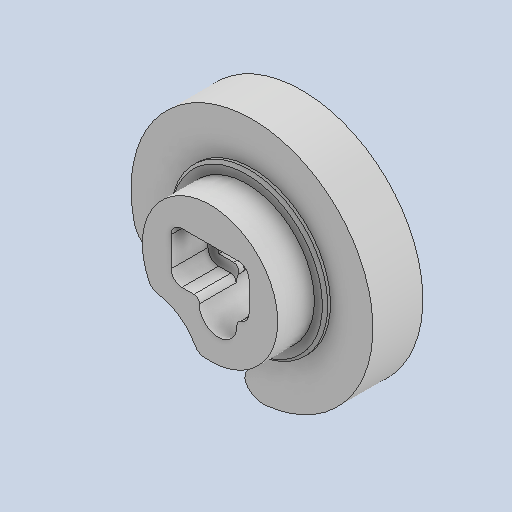
# Autodesk Inventor part: main_wheel_fixator
Saved by Autodesk Inventor 2022 (Build 260153000, 153)
## iProperties
Created: 2024-09-10
Part Number: main_wheel_fixator
Material: Типовые
Document SubType Name: Modeling
Designer: Andrey
Density: 1 g/cm^3
Appearance: По умолчанию
Author: Andrey
Autodesk Inventor part; units mm, degrees
ref_plane "YZ Plane" through (0, 0, 0) normal (1, 0, 0) x (0, 1, 0)
ref_plane "XZ Plane" through (0, 0, 0) normal (0, 1, 0) x (-1, 0, 0)
ref_plane "XY Plane" through (0, 0, 0) normal (0, 0, 1) x (1, 0, 0)
ref_plane "РабПлоскость1" through (-130.0323, -33.3842, -9.2947) normal (0, 0, 1) x (1, 0, 0)
sketch "Эскиз1" plane through (0, 0, 0) normal (0, 0, 1) x (1, 0, 0)
  circle A0 centre (0, 0) radius 22.5
  dimension "d0" = 45
  constraints: 1 centre point, 1 coincident
  measures "d0" diameter of A0
extrude "Выдавливание1" add sketch "Эскиз1" against normal up to surface (9.2947 mm away)
sketch "Эскиз2" plane through (0, 0, 0) normal (0, 0, 1) x (1, 0, 0)
  arc A0 (-12.5314, -17.4431) -> (-12.5619, -14.5867) centre (-11.1467, -16) ccw projected
  circle A1 centre (-11.1467, -16) radius 6.5
  circle A2 centre (-11.1467, -16) radius 9.5
  point P0 (0, 0)
  dimension "d3" = 13
  dimension "d4" = 3
  constraints: 2 centre point, 1 coincident
  measures "d3" diameter of A1
  measures "d4" radial gap between concentric circles of A1 A2
extrude "Выдавливание2" cut sketch "Эскиз2" against normal blind 10 contours A1 | A2
fillet "Сопряжение1" radius 4 2 edges at (-3.9122, -22.1573, -4.6474) (-19.4292, -11.347, -4.6474)
sketch "Эскиз3" plane through (0, 0, 0) normal (0, 0, 1) x (1, 0, 0)
  circle A0 centre (0, 0) radius 12.6
  arc A1 (-21.8671, -5.2989) -> (-15.9551, -7.8067) centre (-17.9796, -4.3569) ccw projected
  arc A2 (-1.795, -17.6717) -> (-15.9551, -7.8067) centre (-11.1467, -16) ccw projected
  arc A3 (-1.795, -17.6717) -> (2.6059, -22.3486) centre (2.1426, -18.3755) ccw projected
  arc A4 (2.6059, -22.3486) -> (-21.8671, -5.2989) centre (0, 0) ccw projected
  line L0 (0, 0) -> (0, -1.1)
  line L1 (5, 3.9) -> (-5, 3.9)
  line L2 (-5, 3.9) -> (-5, -1.1)
  line L3 (-5, -1.1) -> (5, -1.1)
  line L4 (5, -1.1) -> (5, 3.9)
  line L5 (5.25, -1.35) -> (-5.25, -1.35)
  line L6 (-5.25, -1.35) -> (-5.25, 4.15)
  line L7 (-5.25, 4.15) -> (5.25, 4.15)
  line L8 (5.25, 4.15) -> (5.25, -1.35)
  point P0 (-10.7899, -6.5067)
  point P1 (-2.3651, -12.376)
  dimension "d8" = 25.2
  dimension "d35" = 1.1
  dimension "d36" = 10
  dimension "d37" = 5
  dimension "d38" = 0.25
  constraints: 18 end point, 4 parallel, 2 coincident, 2 perpendicular, 1 centre point, 1 horizontal, 1 midpoint, 1 vertical, 3 other
  measures "d8" diameter of A0
  measures "d35" distance of L0.end L0.start
  measures "d36" distance of L3.end L2.end
  measures "d37" distance of L2.end L1.end
  measures "d38" distance between parallel lines of L3 L5
extrude "Выдавливание3" add sketch "Эскиз3" along normal blind 7.8 contours A0 A2 picked at (0.4072, 6.9469)
sketch "Эскиз4" plane through (0, 0, 0) normal (0, 0, 1) x (1, 0, 0)
  arc A0 (-2.3651, -12.376) -> (-10.7899, -6.5067) centre (0, 0) ccw projected
  arc A1 (-1.795, -17.6717) -> (-2.3651, -12.376) centre (-11.1467, -16) ccw projected
  arc A2 (-1.795, -17.6717) -> (2.6059, -22.3486) centre (2.1426, -18.3755) ccw projected
  arc A3 (2.6059, -22.3486) -> (-21.8671, -5.2989) centre (0, 0) ccw projected
  arc A4 (-21.8671, -5.2989) -> (-15.9551, -7.8067) centre (-17.9796, -4.3569) ccw projected
  arc A5 (-10.7899, -6.5067) -> (-15.9551, -7.8067) centre (-11.1467, -16) ccw projected
  circle A6 centre (0, 0) radius 12.6
  circle A7 centre (0, 0) radius 14.6
  point P0 (-1.7671, -14.4927)
  point P1 (-12.9827, -6.6791)
  dimension "d13" = 2
  constraints: 2 centre point, 1 coincident, 1 concentric
  measures "d13" radial gap between concentric circles of A6 A7
extrude "Выдавливание4" add sketch "Эскиз4" along normal blind 1 contours A0 A5 A7 A1
fillet "Сопряжение2" radius 2 4 edges at (-2.3651, -12.376, 4.4) (-1.7671, -14.4927, 0.5) (-10.7899, -6.5067, 4.4) (-12.9827, -6.6791, 0.5)
chamfer "Фаска1" distance 0.5 angle 45 7 edges at (8.3458, 11.9795, 1) (-12.8509, -6.1946, 1) (-11.2228, -6.5003, 1) (-10.3052, -6.5373, 1) (-1.3582, -14.2012, 1) (-2.2091, -12.7799, 1) (-2.5618, -11.932, 1)
sketch "Эскиз5" plane through (0, 0, -9.2947) normal (0, 0, -1) x (-0.8205128, 0.5716281, 0)
  circle A0 centre (-6.9744, -14.6412) radius 1.5
  arc A1 (5.5942, -23.7713) -> (7.8344, -23.1299) centre (6.9744, -24.3588) ccw
  arc A2 (5.5942, -23.7713) -> (5.8702, -23.7046) centre (0, 0) ccw
  spline S0 degree 3 poles (7.0407, -25.2882) (6.986, -25.2268) (6.8766, -25.1041) (6.7176, -24.9155) (6.5628, -24.7236) (6.4128, -24.5278) (6.2678, -24.3283) (6.1284, -24.1248) (6.0175, -23.9518) (5.9319, -23.8114) (5.8908, -23.7402) (5.8702, -23.7046) knots 0 0 0 0 0.125 0.250001 0.375002 0.500002 0.625001 0.75 0.874998 0.937499 1 1 1 1
  arc A3 (7.0407, -25.2882) -> (7.5579, -25.1384) centre (0, 0) ccw
  spline S1 degree 3 poles (7.7014, -23.1745) (7.703, -23.2156) (7.7063, -23.2977) (7.709, -23.4621) (7.7076, -23.6676) (7.6985, -23.9141) (7.6826, -24.1602) (7.6603, -24.4058) (7.632, -24.6508) (7.5984, -24.8952) (7.5714, -25.0573) (7.5579, -25.1384) knots 0 0 0 0 0.062501 0.125002 0.25 0.374999 0.499998 0.624998 0.749999 0.875 1 1 1 1
  arc A4 (7.7014, -23.1745) -> (7.8344, -23.1299) centre (0, 0) ccw
  circle A5 centre (0, -19.5) radius 4.5
  line L0 (-92.3726, 48.2814) -> (-109.8668, 39.9786)
  line L1 (13.2101, -45.7656) -> (-109.8668, 39.9786)
  line L2 (13.2101, -45.7656) -> (14.9372, -26.4783)
  arc A6 (18.1683, -19.9728) -> (14.9372, -26.4783) centre (24.8973, -27.3701) ccw
  arc A7 (18.1683, -19.9728) -> (-19.7633, 18.396) centre (0, 0) ccw
  arc A8 (-26.2813, 17.7001) -> (-19.7633, 18.396) centre (-23.4232, 21.8026) ccw
  line L3 (-26.2813, 17.7001) -> (-36.6493, 24.9232)
  arc A9 (-38.2549, 31.2785) -> (-36.6493, 24.9232) centre (-33.7911, 29.0257) ccw
  arc A10 (-38.2549, 31.2785) -> (-87.3896, 53.5664) centre (-62.359, 43.4437) ccw
  arc A11 (-92.3726, 48.2814) -> (-87.3896, 53.5664) centre (-96.6602, 57.3156) ccw
  circle A12 centre (-4.5825, 16.9412) radius 2.1
  circle A13 centre (10.0321, 14.4) radius 2.1
  circle A14 centre (17.4795, 1.5711) radius 2.1
  circle A15 centre (10.0321, 14.4) radius 3.5
  circle A16 centre (-4.5825, 16.9412) radius 3.5
  circle A17 centre (17.4795, 1.5711) radius 3.5
  circle A18 centre (-52.3269, 57.8437) radius 3.5
  circle A19 centre (-44.8794, 45.0149) radius 3.5
  circle A20 centre (-66.9415, 60.3849) radius 3.5
  circle A21 centre (-63.7005, 38.894) radius 1.5
  circle A22 centre (-3.8031, -2.8349) radius 1.5
  circle A23 centre (-39.8968, 9.209) radius 1.5
  point P0 (0, 0)
  dimension "d20" = 4.2
  dimension "d21" = 4.2
  dimension "d22" = 4.2
  constraints: 3 centre point
  measures "d20" diameter of A12
  measures "d21" diameter of A13
  measures "d22" diameter of A14
extrude "Выдавливание5" cut sketch "Эскиз5" against normal blind 7.5 contours A12 | A13 | A14
sketch "Эскиз6" plane through (0, 0, 7.8) normal (0, 0, 1) x (1, 0, 0)
  circle A0 centre (1.5, -4.5) radius 1.5 projected
  circle A1 centre (1.5, -4.5) radius 1.6
  point P0 (0, 0)
  dimension "d25" = 3.2
  constraints: 1 centre point, 1 coincident
  measures "d25" diameter of A1
extrude "Выдавливание6" cut sketch "Эскиз6" against normal blind 20 contours A0 | A1
sketch "Эскиз7" plane through (0, 0, 7.8) normal (0, 0, 1) x (1, 0, 0)
  circle A0 centre (1.5, -4.5) radius 1.5 projected
  circle A1 centre (1.5, -4.5) radius 3.5
  point P0 (0, 0)
  dimension "d28" = 7
  constraints: 1 centre point, 1 coincident
  measures "d28" diameter of A1
extrude "Выдавливание7" cut sketch "Эскиз7" against normal blind 13 contours A0 | A1
sketch "Эскиз9" plane through (0, 0, 7.8) normal (0, 0, 1) x (1, 0, 0)
  arc A0 (-0.0256, -1.35) -> (3.0256, -1.35) centre (1.5, -4.5) ccw projected
  line L0 (-0.0256, -1.35) -> (-5.25, -1.35) projected
  line L1 (-5.25, -1.35) -> (-5.25, 4.15) projected
  line L2 (-5.25, 4.15) -> (5.25, 4.15) projected
  line L3 (5.25, 4.15) -> (5.25, -1.35) projected
  line L4 (5.25, -1.35) -> (3.0256, -1.35) projected
  arc A1 (-11.3447, -5.4825) -> (-9.8227, -6.5927) centre (-9.544, -4.6122) ccw projected
  arc A2 (-2.7809, -11.4985) -> (-9.8227, -6.5927) centre (-11.1467, -16) ccw projected
  arc A3 (-2.7809, -11.4985) -> (-1.2121, -12.5416) centre (-1.0197, -10.5508) ccw projected
  arc A4 (-1.2121, -12.5416) -> (-11.3447, -5.4825) centre (0, 0) ccw projected
  arc A5 (-3.8784, -3.35) -> (6.8784, -3.35) centre (1.5, -4.5) ccw
  line L5 (-3.8784, -3.35) -> (-7.25, -3.35)
  line L6 (-7.25, -3.35) -> (-7.25, 6.15)
  line L7 (-7.25, 6.15) -> (7.25, 6.15)
  line L8 (7.25, 6.15) -> (7.25, -3.35)
  line L9 (7.25, -3.35) -> (6.8784, -3.35)
  line L10 (7.25, -3.35) -> (-7.25, -3.35)
  point P0 (4.8057, -3.35)
  point P1 (6.8784, -3.35)
  point P2 (-1.8057, -3.35)
  dimension "d39" = 2
  constraints: 12 end point, 2 point on circle, 1 centre point, 1 collinear, 5 other
  measures "d39" distance between parallel lines of L4 L9
extrude "Выдавливание9" cut sketch "Эскиз9" against normal blind 6.85 contours A0 L10 L5 L6 L7 L8 L9 L4 L3 L2 L1 L0
fillet "Сопряжение3" radius 2 4 edges at (7.25, -3.35, 4.375) (-7.25, -3.35, 4.375) (-7.25, 6.15, 4.375) (7.25, 6.15, 4.375)
fillet "Сопряжение4" radius 1 4 edges at (-1.8057, -3.35, 4.375) (4.8057, -3.35, 4.375) (3.0256, -1.35, 0.475) (-0.0256, -1.35, 0.475)
sketch "Эскиз10" plane through (0, 0, 0) normal (0, 0, 1) x (1, 0, 0)
  circle A0 centre (-2.6467, -16) radius 1.5 projected
  circle A1 centre (-19.6467, -16) radius 1.5 projected
  line L0 (55, -39.3) -> (55, -42.3) projected
  line L1 (55, -42.3) -> (47, -42.3) projected
  line L2 (47, -42.3) -> (47, -39.3) projected
  line L3 (47, -39.3) -> (55, -39.3) projected
  line L4 (29, -39.3) -> (29, -42.3) projected
  line L5 (29, -42.3) -> (21, -42.3) projected
  line L6 (21, -42.3) -> (21, -39.3) projected
  line L7 (21, -39.3) -> (29, -39.3) projected
  arc A2 (56, -45.3) -> (59, -42.3) centre (56, -42.3) ccw projected
  line L8 (59, -42.3) -> (59, -31) projected
  arc A3 (60, -30) -> (59, -31) centre (60, -31) ccw projected
  line L9 (117, -30) -> (60, -30) projected
  line L10 (106.6702, -16.2098) -> (117, -30) projected
  arc A4 (105.0053, -7.6609) -> (106.6702, -16.2098) centre (114.6738, -10.2146) ccw projected
  arc A5 (105.0053, -7.6609) -> (46.249, 3.8571) centre (76, 0) ccw projected
  arc A6 (41.2905, -0.5) -> (46.249, 3.8571) centre (41.2905, 4.5) ccw projected
  line L11 (34.7095, -0.5) -> (41.2905, -0.5) projected
  arc A7 (29.751, 3.8571) -> (34.7095, -0.5) centre (34.7095, 4.5) ccw projected
  arc A8 (29.751, 3.8571) -> (-29.0053, -7.6609) centre (0, 0) ccw projected
  arc A9 (-30.6702, -16.2098) -> (-29.0053, -7.6609) centre (-38.6738, -10.2146) ccw projected
  line L12 (-41, -30) -> (-30.6702, -16.2098) projected
  line L13 (16, -30) -> (-41, -30) projected
  arc A10 (17, -31) -> (16, -30) centre (16, -31) ccw projected
  line L14 (17, -31) -> (17, -42.3) projected
  arc A11 (17, -42.3) -> (20, -45.3) centre (20, -42.3) ccw projected
  line L15 (20, -45.3) -> (30.5, -45.3) projected
  line L16 (30.5, -45.3) -> (30.5, -44.1) projected
  arc A12 (31.5, -43.1) -> (30.5, -44.1) centre (31.5, -44.1) ccw projected
  line L17 (31.5, -43.1) -> (44.5, -43.1) projected
  arc A13 (45.5, -44.1) -> (44.5, -43.1) centre (44.5, -44.1) ccw projected
  line L18 (45.5, -44.1) -> (45.5, -45.3) projected
  line L19 (45.5, -45.3) -> (56, -45.3) projected
  circle A14 centre (8.4252, -24) radius 1.5 projected
  circle A15 centre (105.1467, -24) radius 1.5 projected
  circle A16 centre (67.5748, -24) radius 1.5 projected
  circle A17 centre (-29.1467, -24) radius 1.5 projected
  circle A18 centre (38, -15.25) radius 3 projected
  circle A19 centre (74.5, -4.5) radius 1.5 projected
  circle A20 centre (1.5, -4.5) radius 1.5 projected
  circle A21 centre (89.4441, 11.2809) radius 1.5 projected
  circle A22 centre (76, 17.55) radius 1.5 projected
  circle A23 centre (62.5559, 11.2809) radius 1.5 projected
  circle A24 centre (-13.4441, 11.2809) radius 1.5 projected
  circle A25 centre (0, 17.55) radius 1.5 projected
  circle A26 centre (13.4441, 11.2809) radius 1.5 projected
  circle A27 centre (-11.1467, -16) radius 5.6 projected
  circle A28 centre (-2.6467, -16) radius 3
  point P0 (0, 0)
  dimension "d44" = 6
  constraints: 1 centre point, 1 coincident
  measures "d44" diameter of A28
extrude "Выдавливание10" cut sketch "Эскиз10" along normal mid plane 30 contours A0 | A27 A28 | A27 A28 picked at (-5.6085, -16) picked at (-0.1909, -16.3616)
fillet "Сопряжение5" radius 2 2 edges at (-2.1173, -13.0471, -4.3974) (-1.8248, -18.8852, -4.6474)
